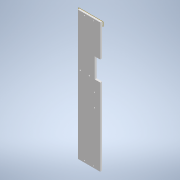
# Autodesk Inventor part: top of metal drivetrain
Saved by Autodesk Inventor 2020 (Build 240168000, 168)
## iProperties
Created: 2020-02-27
Part Number: top of metal drivetrain
Material: Generic
Document SubType Name: Modeling
Designer: jackm
Density: 1 g/cm^3
Appearance: Default
Author: jackm
Autodesk Inventor part; units mm, degrees
ref_plane "YZ Plane" through (0, 0, 0) normal (1, 0, 0) x (0, 1, 0)
ref_plane "XZ Plane" through (0, 0, 0) normal (0, 1, 0) x (-1, 0, 0)
ref_plane "XY Plane" through (0, 0, 0) normal (0, 0, 1) x (1, 0, 0)
ref_plane "Work Plane1" through (0, 0, 0) normal (0, 0, 1) x (1, 0, 0)
sketch "Sketch1" plane through (0, 0, 0) normal (0, 0, 1) x (1, 0, 0)
  line L0 (0, -438.15) -> (0, 12.7) construction
  line L1 (77.6738, 12.7) -> (77.6738, -438.15) construction
  line L2 (0, 12.7) -> (77.6738, 12.7)
  line L3 (0, 12.7) -> (0, -438.15)
  line L4 (0, -438.15) -> (77.6738, -438.15)
  line L5 (77.6738, -438.15) -> (77.6738, 12.7)
  circle A0 centre (54.7859, 6.35) radius 1.7 construction
  arc A1 (22.7012, 8.05) -> (22.9879, 8.05) centre (22.8446, 6.35) ccw construction
  circle A2 centre (54.7859, 6.35) radius 1.7
  circle A3 centre (22.8446, 6.35) radius 1.7
  arc A4 (54.972, -433.5) -> (54.6853, -433.5) centre (54.8286, -431.8) ccw construction
  circle A5 centre (22.8873, -431.8) radius 1.7 construction
  circle A6 centre (54.8286, -431.8) radius 1.7
  circle A7 centre (22.8873, -431.8) radius 1.7
  ellipse E0 centre (57.4571, -254.7292) end of major axis (57.4571, -252.7988) minor radius 1.9304 construction
  ellipse E1 centre (57.4571, -208.0147) end of major axis (57.4571, -206.0843) minor radius 1.9304 construction
  circle A8 centre (57.4571, -208.0147) radius 1.778
  circle A9 centre (57.4571, -254.7292) radius 1.778
  circle A10 centre (40, -166.7445) radius 1.9304 construction
  circle A11 centre (8, -166.7445) radius 1.9304 construction
  circle A12 centre (8, -166.7445) radius 2.25
  circle A13 centre (40, -166.7445) radius 2.25
  line L6 (87.6732, -438.15) -> (87.6732, 12.7) construction
  point P0 (0, 0)
  dimension "d0" = 3.4
  dimension "d1" = 3.4
  dimension "d2" = 3.4
  dimension "d3" = 3.4
  dimension "d4" = 3.556
  dimension "d5" = 3.556
  dimension "d6" = 4.5
  dimension "d7" = 4.5
  constraints: 8 centre point, 8 coincident, 8 end point, 4 perpendicular
  measures "d0" diameter of A2
  measures "d1" diameter of A3
  measures "d2" diameter of A6
  measures "d3" diameter of A7
  measures "d4" diameter of A8
  measures "d5" diameter of A9
  measures "d6" diameter of A12
  measures "d7" diameter of A13
extrude "Extrusion1" add sketch "Sketch1" along normal blind 6.35
sketch "Sketch2" plane through (0, 0, 6.35) normal (0, 0, 1) x (1, 0, 0)
  line L0 (77.6738, -438.15) -> (77.6738, 12.7) projected
  line L1 (77.6738, -99.3902) -> (77.6738, -168.91)
  line L2 (77.6738, -168.91) -> (58.6238, -168.91)
  line L3 (58.6238, -168.91) -> (58.6238, -99.3902)
  line L4 (58.6238, -99.3902) -> (77.6738, -99.3902)
  line L5 (77.6738, 12.7) -> (0, 12.7) projected
  line L6 (0, -438.15) -> (77.6738, -438.15) projected
  point P0 (0, 0)
  dimension "d10" = 19.05
  dimension "d13" = 112.0902
  dimension "d14" = 269.24
  constraints: 8 end point, 3 perpendicular, 2 point on line
  measures "d10" distance of L1.end L2.end
  measures "d13" distance between parallel lines of L5 L4
  measures "d14" distance between parallel lines of L6 L2
extrude "Extrusion2" cut sketch "Sketch2" against normal blind 6.35
body "Solid1"
